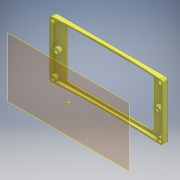
# Autodesk Inventor part: Peça 8
Saved by Autodesk Inventor 2016 (Build 200138000, 138)
## iProperties
Created: 2018-09-27
Part Number: Peça 8
Material: Generic
Document SubType Name: Modeling
Designer: dqm_r
Density: 1 g/cm^3
Appearance: Smooth - Yellow
Author: dqm_r
Autodesk Inventor part; units mm, degrees
ref_plane "YZ Plane" through (0, 0, 0) normal (1, 0, 0) x (0, 1, 0)
ref_plane "XZ Plane" through (0, 0, 0) normal (0, 1, 0) x (-1, 0, 0)
ref_plane "XY Plane" through (0, 0, 0) normal (0, 0, 1) x (1, 0, 0)
sketch "Sketch1" plane through (0, 0, 0) normal (0, 1, 0) x (-1, 0, 0)
  line L0 (-43.8, 22.875) -> (43.8, 22.875)
  line L1 (45.8, 20.875) -> (45.8, -20.875)
  line L2 (43.8, -22.875) -> (-43.8, -22.875)
  line L3 (-45.8, -20.875) -> (-45.8, 20.875)
  line L4 (-35.6, -17.675) -> (-35.6, 17.675)
  line L5 (0, -19.675) -> (-33.6, -19.675)
  line L6 (0, 19.675) -> (33.6, 19.675)
  line L7 (35.6, -17.675) -> (35.6, 17.675)
  line L8 (0, -19.675) -> (33.6, -19.675)
  line L9 (0, 19.675) -> (-33.6, 19.675)
  arc A0 (33.6, -19.675) -> (35.6, -17.675) centre (33.6, -17.675) ccw
  arc A1 (35.6, 17.675) -> (33.6, 19.675) centre (33.6, 17.675) ccw
  arc A2 (-33.6, 19.675) -> (-35.6, 17.675) centre (-33.6, 17.675) ccw
  arc A3 (-35.6, -17.675) -> (-33.6, -19.675) centre (-33.6, -17.675) ccw
  circle A4 centre (-40.7, 0) radius 1.5
  circle A5 centre (40.7, 0) radius 1.5
  arc A6 (43.8, -22.875) -> (45.8, -20.875) centre (43.8, -20.875) ccw
  arc A7 (45.8, 20.875) -> (43.8, 22.875) centre (43.8, 20.875) ccw
  arc A8 (-43.8, 22.875) -> (-45.8, 20.875) centre (-43.8, 20.875) ccw
  arc A9 (-45.8, -20.875) -> (-43.8, -22.875) centre (-43.8, -20.875) ccw
  point P0 (0, 0)
  point P1 (-35.6, -22.875)
  point P2 (-35.6, 22.875)
  point P3 (-45.8, -19.675)
  point P4 (45.8, 19.675)
  point P5 (35.6, -22.875)
  point P6 (35.6, 22.875)
  point P7 (45.8, -19.675)
  point P8 (45.8, -20.875)
  point P9 (43.8, -22.875)
  point P10 (43.8, 22.875)
  point P11 (-45.8, 20.875)
  point P12 (-43.8, 22.875)
  point P13 (-43.8, -22.875)
  constraints: 20 end point, 16 point on circle, 16 tangent, 10 centre point, 10 point on line, 6 equal radius, 3 perpendicular, 2 parallel, 1 horizontal
extrude "Extrusion1" add sketch "Sketch1" against normal blind 4.3
sketch "Sketch3" plane through (-43.8, 0, 22.875) normal (0, 0, 1) x (1, 0, 0)
  arc A0 (89.6, -4.3) -> (-2, -4.3) centre (43.8, -702.7633) ccw
  line L0 (89.6, -4.3) -> (-2, -4.3)
  line L1 (4.6, 0) -> (4.6, -4.3) projected
  point P0 (43.8, 0)
  constraints: 2 end point, 2 point on circle, 1 centre point, 1 perpendicular
extrude "Extrusion3" cut sketch "Sketch3" against normal up to surface (45.75 mm away)
sketch "Sketch5" plane through (0, 0, 0) normal (0, 1, 0) x (1, 0, 0)
  line L0 (45.8, 20.875) -> (45.8, -20.875) projected
  line L1 (-43.8, 22.875) -> (43.8, 22.875) projected
  line L2 (45.8, 22.875) -> (43.4, 22.875)
  line L3 (43.4, 22.875) -> (43.4, 20.475)
  point P0 (0, 0)
  dimension "d22" = 2.4
  dimension "d23" = 2.4
  constraints: 4 end point, 1 perpendicular, 1 point on line
  measures "d22" distance of L2.start L2.end
  measures "d23" distance of L2.end L3.end
hole "Hole1" at (43.4, 0, -20.475) direction (0, -1, 0) diameter 3 end through all countersink diameter 4 countersink angle 90
mirror "Mirror1" about plane through (0, 0, 0) normal (0, 0, 1) of "Hole1"
mirror "Mirror2" about plane through (0, 0, 0) normal (1, 0, 0) of "Hole1", "Mirror1"
shell "Shell1" thickness 1 removed faces 9 at (44.6001, -4.2224, -0.0012) at (-34.9163, -2.4484, -19.1808) at (-33.9143, -2.4126, 19.6502) at (3.7346, -0.9632, -19.675) at (-3.7346, -0.9632, 19.675) at (33.9143, -2.4126, -19.6502) at (35.2356, -2.459, 18.826) at (35.6, -1.2353, -5.8917) at (-35.6, -2.4706, -5.8917)
ref_plane "Work Plane1" through (-41.3288, -34.5, 21.875) normal (0, -1, 0) x (1, 0, 0)
sketch "Sketch6" plane through (-41.3288, -34.5, 21.875) normal (0, -1, 0) x (1, 0, 0)
  point P0 (41.3288, -21.875)
body "Solid1"
